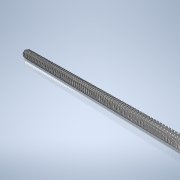
# Autodesk Inventor part: T8x2 (P4) lead screw
Saved by Autodesk Inventor 2020.2 (Build 242310000, 310)
## iProperties
Created: 2020-06-29
Part Number: T8x2 (P4) lead screw
Material: Ogólny
Document SubType Name: Modeling
Designer: Artur Lenart
Density: 1 g/cm^3
Appearance: Stal nierdzewna — jasna
Author: Artur Lenart
Autodesk Inventor part; units mm, degrees
ref_plane "YZ Plane" through (0, 0, 0) normal (1, 0, 0) x (0, 1, 0)
ref_plane "XZ Plane" through (0, 0, 0) normal (0, 1, 0) x (-1, 0, 0)
ref_plane "XY Plane" through (0, 0, 0) normal (0, 0, 1) x (1, 0, 0)
sketch "Szkic1" plane through (0, 0, 0) normal (1, 0, 0) x (0, 1, 0)
  circle A0 centre (0, 0) radius 3
  dimension "d0" = 6
  constraints: 1 centre point, 1 coincident
  measures "d0" diameter of A0
extrude "Wyciągnięcie proste1" add sketch "Szkic1" against normal blind 150
sketch "Szkic2" plane through (0, 0, 0) normal (0, 1, 0) x (-1, 0, 0)
  line L0 (0, -3) -> (-0.8022, -3) construction
  line L1 (0, 0) -> (300, 0) construction
  line L2 (-0.2679, -3) -> (-0.2679, -4) construction
  line L3 (-0.2679, -4) -> (-1, -4)
  line L4 (-1.2679, -3) -> (-1, -4)
  line L5 (-0.2679, -4) -> (0, -3)
  line L6 (-1.2679, -3) -> (0, -3)
  line L7 (0, 3) -> (-0.8022, 3) construction
  line L8 (-1.2679, 3) -> (0, 3)
  line L9 (-0.2679, 3) -> (-0.2679, 4) construction
  line L10 (-0.2679, 4) -> (-1, 4)
  line L11 (-1.2679, 3) -> (-1, 4)
  line L12 (-0.2679, 4) -> (0, 3)
  point P0 (1.2679, -3)
  dimension "d22" = 1
  dimension "d24" = 75
  dimension "d25" = 75
  dimension "d27" = 1
  constraints: 26 end point, 8 symmetric about line, 4 horizontal, 3 point on line, 1 perpendicular
  measures "d22" distance of L2.start L2.end
  measures "d24" angle of L6 L5
  measures "d25" angle of L6 L4
  measures "d27" horizontal distance of L2.end L6.start
coil "Zwój1" sketch "Szkic2" operation add axis through (0, 0, 0) along (-1, 0, 0) pitch 4 turns 37.875 hand right
sketch "Szkic3" plane through (0, 0, 0) normal (0, 1, 0) x (-1, 0, 0)
  line L0 (151.5, 4) -> (150, 4)
  line L1 (150, 4) -> (150, -4)
  line L2 (150, -4) -> (151.5, -4)
  line L3 (151.5, -4) -> (151.5, 4)
  line L4 (150, 3) -> (150, -1.2257) projected
  line L5 (0, 4) -> (-1.5, 4)
  line L6 (-1.5, 4) -> (-1.5, -4)
  line L7 (-1.5, -4) -> (0, -4)
  line L8 (0, -4) -> (0, 4)
  line L9 (0, 0) -> (150, 0) construction
  point P0 (0, 3)
  dimension "d32" = 1.5
  dimension "d33" = 8
  dimension "d34" = 1.5
  dimension "d35" = 8
  dimension "d36" = 8
  dimension "d37" = 8
  constraints: 18 end point, 4 parallel, 3 perpendicular, 3 point on line, 2 horizontal
  measures "d32" distance of L2.end L1.end
  measures "d33" distance of L1.end L0.end
  measures "d34" distance of L7.end L6.end
  measures "d35" distance of L6.end L5.end
  measures "d36" diameter of L0 L9
  measures "d37" diameter of L5 L9
extrude "Wyciągnięcie proste2" cut sketch "Szkic3" along normal mid plane 8
equation "\"d1\" = L"
equation "\"L\" = 150"
